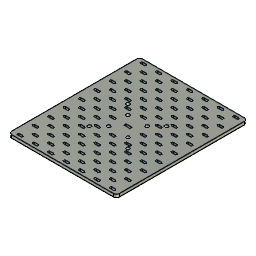
SkadisForUniversalScreenHolder v3 (Autodesk Fusion 360 design; units mm, degrees)
Autodesk Fusion 360 part; units mm, degrees
(part 1 of 2)
sketch "Sketch1" plane through (0, 0, 0) normal (0, 0, 1) x (1, 0, 0)
  line L0 (8, 0) -> (272, 0)
  line L1 (280, 8) -> (280, 332)
  line L2 (272, 340) -> (8, 340)
  line L3 (0, 332) -> (0, 8)
  arc A0 (8, 340) -> (0, 332) centre (8, 332) ccw
  arc A1 (280, 332) -> (272, 340) centre (272, 332) ccw
  arc A2 (272, 0) -> (280, 8) centre (272, 8) ccw
  arc A3 (0, 8) -> (8, 0) centre (8, 8) ccw
  line L4 (8, 8) -> (272, 332) construction
  line L5 (8, 332) -> (272, 8) construction
  line L6 (190, 220) -> (90, 220) construction
  line L7 (90, 220) -> (90, 120) construction
  line L8 (90, 120) -> (190, 120) construction
  line L9 (190, 120) -> (190, 220) construction
  line L10 (190, 220) -> (90, 120) construction
  line L11 (90, 220) -> (190, 120) construction
  line L12 (165, 195) -> (115, 195) construction
  line L13 (115, 195) -> (115, 145) construction
  line L14 (115, 145) -> (165, 145) construction
  line L15 (165, 145) -> (165, 195) construction
  line L16 (165, 195) -> (115, 145) construction
  line L17 (115, 195) -> (165, 145) construction
  circle A4 centre (115, 195) radius 4.5
  circle A5 centre (165, 195) radius 4.5
  circle A6 centre (165, 145) radius 4.5
  circle A7 centre (115, 145) radius 4.5
  circle A8 centre (190, 120) radius 4.5
  circle A9 centre (90, 120) radius 4.5
  circle A10 centre (90, 220) radius 4.5
  circle A11 centre (190, 220) radius 4.5
  point P0 (280, 0)
  point P1 (0, 340)
  point P2 (140, 170)
  point P3 (140, 170)
  dimension "d1" = 280
  dimension "d2" = 340
  dimension "d3" = 8
  dimension "d4" = 100
  dimension "d5" = 100
  dimension "d6" = 50
  dimension "d7" = 50
  dimension "d10" = 9
  dimension "d11" = 9
  dimension "d12" = 9
  dimension "d13" = 9
  dimension "d14" = 9
  dimension "d15" = 9
  dimension "d16" = 9
  dimension "d17" = 9
  constraint horizontal L0
  constraint vertical L1
  constraint horizontal L2
  constraint vertical L3
  constraint coincident P1 L3
  constraint coincident P1 L2
  constraint tangent L3 A0
  constraint tangent L2 A0
  constraint tangent L2 A1
  constraint tangent L1 A1
  constraint equal A0 A1
  constraint coincident P0 L1
  constraint coincident P0 L0
  constraint tangent L1 A2
  constraint tangent L0 A2
  constraint equal A0 A2
  constraint coincident origin L0
  constraint coincident origin L3
  constraint tangent L0 A3
  constraint tangent L3 A3
  constraint equal A0 A3
  constraint coincident A3.centre L4.start
  constraint coincident A1.centre L4.end
  constraint coincident A0.centre L5.start
  constraint coincident A2.centre L5.end
  constraint horizontal L6
  constraint perpendicular L6 L7
  constraint parallel L6 L8
  constraint parallel L7 L9
  constraint coincident L10 P3
  constraint coincident L11 P3
  constraint midpoint L4 P3
  constraint horizontal L12
  constraint perpendicular L12 L13
  constraint parallel L12 L14
  constraint parallel L13 L15
  constraint coincident L16 P3
  constraint coincident L17 P3
  constraint coincident P3 P2
  constraint coincident L12.end L13.start
  constraint coincident L12.start L15.end
  constraint coincident L14.end L15.start
  constraint coincident L13.end L14.start
  constraint coincident L8.end L9.start
  constraint coincident L7.end L8.start
  constraint coincident L6.end L7.start
  constraint coincident L6.start L9.end
  constraint equal A5 A11
  constraint equal A5 A6
  constraint equal A6 A7
  constraint equal A7 A10
  constraint equal A9 A10
  constraint equal A8 A9
  measures "d1" distance of origin P0
  measures "d2" distance of origin P1
  measures "d3" radius of A0
  measures "d4" distance of L7.end L8.end
  measures "d5" distance of L6.end L7.end
  measures "d6" distance of L13.end L14.end
  measures "d7" distance of L12.end L13.end
  measures "d10" diameter of A10
  measures "d11" diameter of A11
  measures "d12" diameter of A5
  measures "d13" diameter of A6
  measures "d14" diameter of A8
  measures "d15" diameter of A7
  measures "d16" diameter of A9
  measures "d17" diameter of A4
extrude "Extrude1" add sketch "Sketch1" along normal blind 8
sketch "Sketch2" plane through (0, 0, 8) normal (0, 0, 1) x (-1, 0, 0)
  circle A0 centre (-165, -145) radius 4.5
  circle A1 centre (-90, -120) radius 4.5
  circle A2 centre (-165, -195) radius 4.5
  circle A3 centre (-190, -120) radius 4.5
  circle A4 centre (-115, -145) radius 4.5
  circle A5 centre (-190, -220) radius 4.5
  circle A6 centre (-90, -220) radius 4.5
  circle A7 centre (-115, -195) radius 4.5
  line L0 (-147.5, -167.5) -> (-132.5, -167.5)
  line L1 (-132.5, -167.5) -> (-132.5, -172.5)
  line L2 (-132.5, -172.5) -> (-147.5, -172.5)
  line L3 (-147.5, -172.5) -> (-147.5, -167.5)
  line L4 (-147.5, -167.5) -> (-132.5, -172.5) construction
  line L5 (-132.5, -167.5) -> (-147.5, -172.5) construction
  line L6 (-135, -167.5) -> (-145, -167.5)
  arc A8 (-145, -167.5) -> (-145, -172.5) centre (-145, -170) ccw
  line L7 (-145, -172.5) -> (-135, -172.5)
  arc A9 (-135, -172.5) -> (-135, -167.5) centre (-135, -170) ccw
  line L8 (-132.5, -170) -> (-147.5, -170) construction
  arc A10 (-255, -332.5) -> (-255, -327.5) centre (-255, -330) ccw
  line L9 (-255, -327.5) -> (-265, -327.5)
  arc A11 (-265, -327.5) -> (-265, -332.5) centre (-265, -330) ccw
  line L10 (-265, -332.5) -> (-255, -332.5)
  arc A12 (-215, -332.5) -> (-215, -327.5) centre (-215, -330) ccw
  line L11 (-215, -327.5) -> (-225, -327.5)
  arc A13 (-225, -327.5) -> (-225, -332.5) centre (-225, -330) ccw
  line L12 (-225, -332.5) -> (-215, -332.5)
  arc A14 (-175, -332.5) -> (-175, -327.5) centre (-175, -330) ccw
  line L13 (-175, -327.5) -> (-185, -327.5)
  arc A15 (-185, -327.5) -> (-185, -332.5) centre (-185, -330) ccw
  line L14 (-185, -332.5) -> (-175, -332.5)
  arc A16 (-135, -332.5) -> (-135, -327.5) centre (-135, -330) ccw
  line L15 (-135, -327.5) -> (-145, -327.5)
  arc A17 (-145, -327.5) -> (-145, -332.5) centre (-145, -330) ccw
  line L16 (-145, -332.5) -> (-135, -332.5)
  arc A18 (-95, -332.5) -> (-95, -327.5) centre (-95, -330) ccw
  line L17 (-95, -327.5) -> (-105, -327.5)
  arc A19 (-105, -327.5) -> (-105, -332.5) centre (-105, -330) ccw
  line L18 (-105, -332.5) -> (-95, -332.5)
  arc A20 (-55, -332.5) -> (-55, -327.5) centre (-55, -330) ccw
  line L19 (-55, -327.5) -> (-65, -327.5)
  arc A21 (-65, -327.5) -> (-65, -332.5) centre (-65, -330) ccw
  line L20 (-65, -332.5) -> (-55, -332.5)
  arc A22 (-15, -332.5) -> (-15, -327.5) centre (-15, -330) ccw
  line L21 (-15, -327.5) -> (-25, -327.5)
  arc A23 (-25, -327.5) -> (-25, -332.5) centre (-25, -330) ccw
  line L22 (-25, -332.5) -> (-15, -332.5)
  arc A24 (-255, -292.5) -> (-255, -287.5) centre (-255, -290) ccw
  line L23 (-255, -287.5) -> (-265, -287.5)
  arc A25 (-265, -287.5) -> (-265, -292.5) centre (-265, -290) ccw
  line L24 (-265, -292.5) -> (-255, -292.5)
  arc A26 (-215, -292.5) -> (-215, -287.5) centre (-215, -290) ccw
  line L25 (-215, -287.5) -> (-225, -287.5)
  arc A27 (-225, -287.5) -> (-225, -292.5) centre (-225, -290) ccw
  line L26 (-225, -292.5) -> (-215, -292.5)
  arc A28 (-175, -292.5) -> (-175, -287.5) centre (-175, -290) ccw
  line L27 (-175, -287.5) -> (-185, -287.5)
  arc A29 (-185, -287.5) -> (-185, -292.5) centre (-185, -290) ccw
  line L28 (-185, -292.5) -> (-175, -292.5)
  arc A30 (-135, -292.5) -> (-135, -287.5) centre (-135, -290) ccw
  line L29 (-135, -287.5) -> (-145, -287.5)
  arc A31 (-145, -287.5) -> (-145, -292.5) centre (-145, -290) ccw
  line L30 (-145, -292.5) -> (-135, -292.5)
  arc A32 (-95, -292.5) -> (-95, -287.5) centre (-95, -290) ccw
  line L31 (-95, -287.5) -> (-105, -287.5)
  arc A33 (-105, -287.5) -> (-105, -292.5) centre (-105, -290) ccw
  line L32 (-105, -292.5) -> (-95, -292.5)
  arc A34 (-55, -292.5) -> (-55, -287.5) centre (-55, -290) ccw
  line L33 (-55, -287.5) -> (-65, -287.5)
  arc A35 (-65, -287.5) -> (-65, -292.5) centre (-65, -290) ccw
  line L34 (-65, -292.5) -> (-55, -292.5)
  arc A36 (-15, -292.5) -> (-15, -287.5) centre (-15, -290) ccw
  line L35 (-15, -287.5) -> (-25, -287.5)
  arc A37 (-25, -287.5) -> (-25, -292.5) centre (-25, -290) ccw
  line L36 (-25, -292.5) -> (-15, -292.5)
  arc A38 (-255, -252.5) -> (-255, -247.5) centre (-255, -250) ccw
  line L37 (-255, -247.5) -> (-265, -247.5)
  arc A39 (-265, -247.5) -> (-265, -252.5) centre (-265, -250) ccw
  line L38 (-265, -252.5) -> (-255, -252.5)
  arc A40 (-215, -252.5) -> (-215, -247.5) centre (-215, -250) ccw
  line L39 (-215, -247.5) -> (-225, -247.5)
  arc A41 (-225, -247.5) -> (-225, -252.5) centre (-225, -250) ccw
  line L40 (-225, -252.5) -> (-215, -252.5)
  arc A42 (-175, -252.5) -> (-175, -247.5) centre (-175, -250) ccw
  line L41 (-175, -247.5) -> (-185, -247.5)
  arc A43 (-185, -247.5) -> (-185, -252.5) centre (-185, -250) ccw
  line L42 (-185, -252.5) -> (-175, -252.5)
  arc A44 (-135, -252.5) -> (-135, -247.5) centre (-135, -250) ccw
  line L43 (-135, -247.5) -> (-145, -247.5)
  arc A45 (-145, -247.5) -> (-145, -252.5) centre (-145, -250) ccw
  line L44 (-145, -252.5) -> (-135, -252.5)
  arc A46 (-95, -252.5) -> (-95, -247.5) centre (-95, -250) ccw
  line L45 (-95, -247.5) -> (-105, -247.5)
  arc A47 (-105, -247.5) -> (-105, -252.5) centre (-105, -250) ccw
  line L46 (-105, -252.5) -> (-95, -252.5)
  arc A48 (-55, -252.5) -> (-55, -247.5) centre (-55, -250) ccw
  line L47 (-55, -247.5) -> (-65, -247.5)
  arc A49 (-65, -247.5) -> (-65, -252.5) centre (-65, -250) ccw
  line L48 (-65, -252.5) -> (-55, -252.5)
  arc A50 (-15, -252.5) -> (-15, -247.5) centre (-15, -250) ccw
  line L49 (-15, -247.5) -> (-25, -247.5)
  arc A51 (-25, -247.5) -> (-25, -252.5) centre (-25, -250) ccw
  line L50 (-25, -252.5) -> (-15, -252.5)
  arc A52 (-255, -212.5) -> (-255, -207.5) centre (-255, -210) ccw
  line L51 (-255, -207.5) -> (-265, -207.5)
  arc A53 (-265, -207.5) -> (-265, -212.5) centre (-265, -210) ccw
  line L52 (-265, -212.5) -> (-255, -212.5)
  arc A54 (-215, -212.5) -> (-215, -207.5) centre (-215, -210) ccw
  line L53 (-215, -207.5) -> (-225, -207.5)
  arc A55 (-225, -207.5) -> (-225, -212.5) centre (-225, -210) ccw
  line L54 (-225, -212.5) -> (-215, -212.5)
  arc A56 (-175, -212.5) -> (-175, -207.5) centre (-175, -210) ccw
  line L55 (-175, -207.5) -> (-185, -207.5)
  arc A57 (-185, -207.5) -> (-185, -212.5) centre (-185, -210) ccw
  line L56 (-185, -212.5) -> (-175, -212.5)
  arc A58 (-135, -212.5) -> (-135, -207.5) centre (-135, -210) ccw
  line L57 (-135, -207.5) -> (-145, -207.5)
  arc A59 (-145, -207.5) -> (-145, -212.5) centre (-145, -210) ccw
  line L58 (-145, -212.5) -> (-135, -212.5)
  arc A60 (-95, -212.5) -> (-95, -207.5) centre (-95, -210) ccw
  line L59 (-95, -207.5) -> (-105, -207.5)
  arc A61 (-105, -207.5) -> (-105, -212.5) centre (-105, -210) ccw
  line L60 (-105, -212.5) -> (-95, -212.5)
  arc A62 (-55, -212.5) -> (-55, -207.5) centre (-55, -210) ccw
  line L61 (-55, -207.5) -> (-65, -207.5)
  arc A63 (-65, -207.5) -> (-65, -212.5) centre (-65, -210) ccw
  line L62 (-65, -212.5) -> (-55, -212.5)
  arc A64 (-15, -212.5) -> (-15, -207.5) centre (-15, -210) ccw
  line L63 (-15, -207.5) -> (-25, -207.5)
  arc A65 (-25, -207.5) -> (-25, -212.5) centre (-25, -210) ccw
  line L64 (-25, -212.5) -> (-15, -212.5)
  arc A66 (-255, -172.5) -> (-255, -167.5) centre (-255, -170) ccw
  line L65 (-255, -167.5) -> (-265, -167.5)
  arc A67 (-265, -167.5) -> (-265, -172.5) centre (-265, -170) ccw
  line L66 (-265, -172.5) -> (-255, -172.5)
  arc A68 (-215, -172.5) -> (-215, -167.5) centre (-215, -170) ccw
  line L67 (-215, -167.5) -> (-225, -167.5)
  arc A69 (-225, -167.5) -> (-225, -172.5) centre (-225, -170) ccw
  line L68 (-225, -172.5) -> (-215, -172.5)
  arc A70 (-175, -172.5) -> (-175, -167.5) centre (-175, -170) ccw
  line L69 (-175, -167.5) -> (-185, -167.5)
  arc A71 (-185, -167.5) -> (-185, -172.5) centre (-185, -170) ccw
  line L70 (-185, -172.5) -> (-175, -172.5)
  arc A72 (-95, -172.5) -> (-95, -167.5) centre (-95, -170) ccw
  line L71 (-95, -167.5) -> (-105, -167.5)
  arc A73 (-105, -167.5) -> (-105, -172.5) centre (-105, -170) ccw
  line L72 (-105, -172.5) -> (-95, -172.5)
  arc A74 (-55, -172.5) -> (-55, -167.5) centre (-55, -170) ccw
  line L73 (-55, -167.5) -> (-65, -167.5)
  arc A75 (-65, -167.5) -> (-65, -172.5) centre (-65, -170) ccw
  line L74 (-65, -172.5) -> (-55, -172.5)
  arc A76 (-15, -172.5) -> (-15, -167.5) centre (-15, -170) ccw
  line L75 (-15, -167.5) -> (-25, -167.5)
  arc A77 (-25, -167.5) -> (-25, -172.5) centre (-25, -170) ccw
  line L76 (-25, -172.5) -> (-15, -172.5)
  arc A78 (-255, -132.5) -> (-255, -127.5) centre (-255, -130) ccw
  line L77 (-255, -127.5) -> (-265, -127.5)
  arc A79 (-265, -127.5) -> (-265, -132.5) centre (-265, -130) ccw
  line L78 (-265, -132.5) -> (-255, -132.5)
  arc A80 (-215, -132.5) -> (-215, -127.5) centre (-215, -130) ccw
  line L79 (-215, -127.5) -> (-225, -127.5)
  arc A81 (-225, -127.5) -> (-225, -132.5) centre (-225, -130) ccw
  line L80 (-225, -132.5) -> (-215, -132.5)
  arc A82 (-175, -132.5) -> (-175, -127.5) centre (-175, -130) ccw
  line L81 (-175, -127.5) -> (-185, -127.5)
  arc A83 (-185, -127.5) -> (-185, -132.5) centre (-185, -130) ccw
  line L82 (-185, -132.5) -> (-175, -132.5)
  arc A84 (-135, -132.5) -> (-135, -127.5) centre (-135, -130) ccw
  line L83 (-135, -127.5) -> (-145, -127.5)
  arc A85 (-145, -127.5) -> (-145, -132.5) centre (-145, -130) ccw
  line L84 (-145, -132.5) -> (-135, -132.5)
  arc A86 (-95, -132.5) -> (-95, -127.5) centre (-95, -130) ccw
  line L85 (-95, -127.5) -> (-105, -127.5)
  arc A87 (-105, -127.5) -> (-105, -132.5) centre (-105, -130) ccw
  line L86 (-105, -132.5) -> (-95, -132.5)
  arc A88 (-55, -132.5) -> (-55, -127.5) centre (-55, -130) ccw
  line L87 (-55, -127.5) -> (-65, -127.5)
  arc A89 (-65, -127.5) -> (-65, -132.5) centre (-65, -130) ccw
  line L88 (-65, -132.5) -> (-55, -132.5)
  arc A90 (-15, -132.5) -> (-15, -127.5) centre (-15, -130) ccw
  line L89 (-15, -127.5) -> (-25, -127.5)
  arc A91 (-25, -127.5) -> (-25, -132.5) centre (-25, -130) ccw
  line L90 (-25, -132.5) -> (-15, -132.5)
  arc A92 (-255, -92.5) -> (-255, -87.5) centre (-255, -90) ccw
  line L91 (-255, -87.5) -> (-265, -87.5)
  arc A93 (-265, -87.5) -> (-265, -92.5) centre (-265, -90) ccw
  line L92 (-265, -92.5) -> (-255, -92.5)
  arc A94 (-215, -92.5) -> (-215, -87.5) centre (-215, -90) ccw
  line L93 (-215, -87.5) -> (-225, -87.5)
  arc A95 (-225, -87.5) -> (-225, -92.5) centre (-225, -90) ccw
  line L94 (-225, -92.5) -> (-215, -92.5)
  arc A96 (-175, -92.5) -> (-175, -87.5) centre (-175, -90) ccw
  line L95 (-175, -87.5) -> (-185, -87.5)
  arc A97 (-185, -87.5) -> (-185, -92.5) centre (-185, -90) ccw
  line L96 (-185, -92.5) -> (-175, -92.5)
  arc A98 (-135, -92.5) -> (-135, -87.5) centre (-135, -90) ccw
  line L97 (-135, -87.5) -> (-145, -87.5)
  arc A99 (-145, -87.5) -> (-145, -92.5) centre (-145, -90) ccw
  line L98 (-145, -92.5) -> (-135, -92.5)
  arc A100 (-95, -92.5) -> (-95, -87.5) centre (-95, -90) ccw
  line L99 (-95, -87.5) -> (-105, -87.5)
  arc A101 (-105, -87.5) -> (-105, -92.5) centre (-105, -90) ccw
  line L100 (-105, -92.5) -> (-95, -92.5)
  arc A102 (-55, -92.5) -> (-55, -87.5) centre (-55, -90) ccw
  line L101 (-55, -87.5) -> (-65, -87.5)
  arc A103 (-65, -87.5) -> (-65, -92.5) centre (-65, -90) ccw
  line L102 (-65, -92.5) -> (-55, -92.5)
  arc A104 (-15, -92.5) -> (-15, -87.5) centre (-15, -90) ccw
  line L103 (-15, -87.5) -> (-25, -87.5)
  arc A105 (-25, -87.5) -> (-25, -92.5) centre (-25, -90) ccw
  line L104 (-25, -92.5) -> (-15, -92.5)
  arc A106 (-255, -52.5) -> (-255, -47.5) centre (-255, -50) ccw
  line L105 (-255, -47.5) -> (-265, -47.5)
  arc A107 (-265, -47.5) -> (-265, -52.5) centre (-265, -50) ccw
  line L106 (-265, -52.5) -> (-255, -52.5)
  arc A108 (-215, -52.5) -> (-215, -47.5) centre (-215, -50) ccw
  line L107 (-215, -47.5) -> (-225, -47.5)
  arc A109 (-225, -47.5) -> (-225, -52.5) centre (-225, -50) ccw
  line L108 (-225, -52.5) -> (-215, -52.5)
  arc A110 (-175, -52.5) -> (-175, -47.5) centre (-175, -50) ccw
  line L109 (-175, -47.5) -> (-185, -47.5)
  arc A111 (-185, -47.5) -> (-185, -52.5) centre (-185, -50) ccw
  line L110 (-185, -52.5) -> (-175, -52.5)
  arc A112 (-135, -52.5) -> (-135, -47.5) centre (-135, -50) ccw
  line L111 (-135, -47.5) -> (-145, -47.5)
  arc A113 (-145, -47.5) -> (-145, -52.5) centre (-145, -50) ccw
  line L112 (-145, -52.5) -> (-135, -52.5)
  arc A114 (-95, -52.5) -> (-95, -47.5) centre (-95, -50) ccw
  line L113 (-95, -47.5) -> (-105, -47.5)
  arc A115 (-105, -47.5) -> (-105, -52.5) centre (-105, -50) ccw
  line L114 (-105, -52.5) -> (-95, -52.5)
  arc A116 (-55, -52.5) -> (-55, -47.5) centre (-55, -50) ccw
  line L115 (-55, -47.5) -> (-65, -47.5)
  arc A117 (-65, -47.5) -> (-65, -52.5) centre (-65, -50) ccw
  line L116 (-65, -52.5) -> (-55, -52.5)
  arc A118 (-15, -52.5) -> (-15, -47.5) centre (-15, -50) ccw
  line L117 (-15, -47.5) -> (-25, -47.5)
  arc A119 (-25, -47.5) -> (-25, -52.5) centre (-25, -50) ccw
  line L118 (-25, -52.5) -> (-15, -52.5)
  arc A120 (-255, -12.5) -> (-255, -7.5) centre (-255, -10) ccw
  line L119 (-255, -7.5) -> (-265, -7.5)
  arc A121 (-265, -7.5) -> (-265, -12.5) centre (-265, -10) ccw
  line L120 (-265, -12.5) -> (-255, -12.5)
  arc A122 (-215, -12.5) -> (-215, -7.5) centre (-215, -10) ccw
  line L121 (-215, -7.5) -> (-225, -7.5)
  arc A123 (-225, -7.5) -> (-225, -12.5) centre (-225, -10) ccw
  line L122 (-225, -12.5) -> (-215, -12.5)
  arc A124 (-175, -12.5) -> (-175, -7.5) centre (-175, -10) ccw
  line L123 (-175, -7.5) -> (-185, -7.5)
  arc A125 (-185, -7.5) -> (-185, -12.5) centre (-185, -10) ccw
  line L124 (-185, -12.5) -> (-175, -12.5)
  arc A126 (-135, -12.5) -> (-135, -7.5) centre (-135, -10) ccw
  line L125 (-135, -7.5) -> (-145, -7.5)
  arc A127 (-145, -7.5) -> (-145, -12.5) centre (-145, -10) ccw
  line L126 (-145, -12.5) -> (-135, -12.5)
  arc A128 (-95, -12.5) -> (-95, -7.5) centre (-95, -10) ccw
  line L127 (-95, -7.5) -> (-105, -7.5)
  arc A129 (-105, -7.5) -> (-105, -12.5) centre (-105, -10) ccw
  line L128 (-105, -12.5) -> (-95, -12.5)
  arc A130 (-55, -12.5) -> (-55, -7.5) centre (-55, -10) ccw
  line L129 (-55, -7.5) -> (-65, -7.5)
  arc A131 (-65, -7.5) -> (-65, -12.5) centre (-65, -10) ccw
  line L130 (-65, -12.5) -> (-55, -12.5)
  arc A132 (-15, -12.5) -> (-15, -7.5) centre (-15, -10) ccw
  line L131 (-15, -7.5) -> (-25, -7.5)
  arc A133 (-25, -7.5) -> (-25, -12.5) centre (-25, -10) ccw
  line L132 (-25, -12.5) -> (-15, -12.5)
  line L133 (-35, -27.5) -> (-45, -27.5)
  arc A134 (-45, -27.5) -> (-45, -32.5) centre (-45, -30) ccw
  line L134 (-45, -32.5) -> (-35, -32.5)
  arc A135 (-35, -32.5) -> (-35, -27.5) centre (-35, -30) ccw
  line L135 (-85, -32.5) -> (-75, -32.5)
  arc A136 (-75, -32.5) -> (-75, -27.5) centre (-75, -30) ccw
  line L136 (-75, -27.5) -> (-85, -27.5)
  arc A137 (-85, -27.5) -> (-85, -32.5) centre (-85, -30) ccw
  line L137 (-125, -32.5) -> (-115, -32.5)
  arc A138 (-115, -32.5) -> (-115, -27.5) centre (-115, -30) ccw
  line L138 (-115, -27.5) -> (-125, -27.5)
  arc A139 (-125, -27.5) -> (-125, -32.5) centre (-125, -30) ccw
  line L139 (-165, -32.5) -> (-155, -32.5)
  arc A140 (-155, -32.5) -> (-155, -27.5) centre (-155, -30) ccw
  line L140 (-155, -27.5) -> (-165, -27.5)
  arc A141 (-165, -27.5) -> (-165, -32.5) centre (-165, -30) ccw
  line L141 (-205, -32.5) -> (-195, -32.5)
  arc A142 (-195, -32.5) -> (-195, -27.5) centre (-195, -30) ccw
  line L142 (-195, -27.5) -> (-205, -27.5)
  arc A143 (-205, -27.5) -> (-205, -32.5) centre (-205, -30) ccw
  line L143 (-245, -32.5) -> (-235, -32.5)
  arc A144 (-235, -32.5) -> (-235, -27.5) centre (-235, -30) ccw
  line L144 (-235, -27.5) -> (-245, -27.5)
  arc A145 (-245, -27.5) -> (-245, -32.5) centre (-245, -30) ccw
  line L145 (-45, -72.5) -> (-35, -72.5)
  arc A146 (-35, -72.5) -> (-35, -67.5) centre (-35, -70) ccw
  line L146 (-35, -67.5) -> (-45, -67.5)
  arc A147 (-45, -67.5) -> (-45, -72.5) centre (-45, -70) ccw
  line L147 (-85, -72.5) -> (-75, -72.5)
  arc A148 (-75, -72.5) -> (-75, -67.5) centre (-75, -70) ccw
  line L148 (-75, -67.5) -> (-85, -67.5)
  arc A149 (-85, -67.5) -> (-85, -72.5) centre (-85, -70) ccw
  line L149 (-125, -72.5) -> (-115, -72.5)
  arc A150 (-115, -72.5) -> (-115, -67.5) centre (-115, -70) ccw
  line L150 (-115, -67.5) -> (-125, -67.5)
  arc A151 (-125, -67.5) -> (-125, -72.5) centre (-125, -70) ccw
  line L151 (-165, -72.5) -> (-155, -72.5)
  arc A152 (-155, -72.5) -> (-155, -67.5) centre (-155, -70) ccw
  line L152 (-155, -67.5) -> (-165, -67.5)
  arc A153 (-165, -67.5) -> (-165, -72.5) centre (-165, -70) ccw
  line L153 (-205, -72.5) -> (-195, -72.5)
  arc A154 (-195, -72.5) -> (-195, -67.5) centre (-195, -70) ccw
  line L154 (-195, -67.5) -> (-205, -67.5)
  arc A155 (-205, -67.5) -> (-205, -72.5) centre (-205, -70) ccw
  line L155 (-245, -72.5) -> (-235, -72.5)
  arc A156 (-235, -72.5) -> (-235, -67.5) centre (-235, -70) ccw
  line L156 (-235, -67.5) -> (-245, -67.5)
  arc A157 (-245, -67.5) -> (-245, -72.5) centre (-245, -70) ccw
  line L157 (-45, -112.5) -> (-35, -112.5)
  arc A158 (-35, -112.5) -> (-35, -107.5) centre (-35, -110) ccw
  line L158 (-35, -107.5) -> (-45, -107.5)
  arc A159 (-45, -107.5) -> (-45, -112.5) centre (-45, -110) ccw
  line L159 (-85, -112.5) -> (-75, -112.5)
  arc A160 (-75, -112.5) -> (-75, -107.5) centre (-75, -110) ccw
  line L160 (-75, -107.5) -> (-85, -107.5)
  arc A161 (-85, -107.5) -> (-85, -112.5) centre (-85, -110) ccw
  line L161 (-125, -112.5) -> (-115, -112.5)
  arc A162 (-115, -112.5) -> (-115, -107.5) centre (-115, -110) ccw
  line L162 (-115, -107.5) -> (-125, -107.5)
  arc A163 (-125, -107.5) -> (-125, -112.5) centre (-125, -110) ccw
  line L163 (-165, -112.5) -> (-155, -112.5)
  arc A164 (-155, -112.5) -> (-155, -107.5) centre (-155, -110) ccw
  line L164 (-155, -107.5) -> (-165, -107.5)
  arc A165 (-165, -107.5) -> (-165, -112.5) centre (-165, -110) ccw
  line L165 (-205, -112.5) -> (-195, -112.5)
  arc A166 (-195, -112.5) -> (-195, -107.5) centre (-195, -110) ccw
  line L166 (-195, -107.5) -> (-205, -107.5)
  arc A167 (-205, -107.5) -> (-205, -112.5) centre (-205, -110) ccw
  line L167 (-245, -112.5) -> (-235, -112.5)
  arc A168 (-235, -112.5) -> (-235, -107.5) centre (-235, -110) ccw
  line L168 (-235, -107.5) -> (-245, -107.5)
  arc A169 (-245, -107.5) -> (-245, -112.5) centre (-245, -110) ccw
  line L169 (-45, -152.5) -> (-35, -152.5)
  arc A170 (-35, -152.5) -> (-35, -147.5) centre (-35, -150) ccw
  line L170 (-35, -147.5) -> (-45, -147.5)
  arc A171 (-45, -147.5) -> (-45, -152.5) centre (-45, -150) ccw
  line L171 (-85, -152.5) -> (-75, -152.5)
  arc A172 (-75, -152.5) -> (-75, -147.5) centre (-75, -150) ccw
  line L172 (-75, -147.5) -> (-85, -147.5)
  arc A173 (-85, -147.5) -> (-85, -152.5) centre (-85, -150) ccw
  line L173 (-205, -152.5) -> (-195, -152.5)
  arc A174 (-195, -152.5) -> (-195, -147.5) centre (-195, -150) ccw
  line L174 (-195, -147.5) -> (-205, -147.5)
  arc A175 (-205, -147.5) -> (-205, -152.5) centre (-205, -150) ccw
  line L175 (-245, -152.5) -> (-235, -152.5)
  arc A176 (-235, -152.5) -> (-235, -147.5) centre (-235, -150) ccw
  line L176 (-235, -147.5) -> (-245, -147.5)
  arc A177 (-245, -147.5) -> (-245, -152.5) centre (-245, -150) ccw
  line L177 (-45, -192.5) -> (-35, -192.5)
  arc A178 (-35, -192.5) -> (-35, -187.5) centre (-35, -190) ccw
  line L178 (-35, -187.5) -> (-45, -187.5)
  arc A179 (-45, -187.5) -> (-45, -192.5) centre (-45, -190) ccw
  line L179 (-85, -192.5) -> (-75, -192.5)
  arc A180 (-75, -192.5) -> (-75, -187.5) centre (-75, -190) ccw
  line L180 (-75, -187.5) -> (-85, -187.5)
  arc A181 (-85, -187.5) -> (-85, -192.5) centre (-85, -190) ccw
  line L181 (-205, -192.5) -> (-195, -192.5)
  arc A182 (-195, -192.5) -> (-195, -187.5) centre (-195, -190) ccw
  line L182 (-195, -187.5) -> (-205, -187.5)
  arc A183 (-205, -187.5) -> (-205, -192.5) centre (-205, -190) ccw
  line L183 (-245, -192.5) -> (-235, -192.5)
  arc A184 (-235, -192.5) -> (-235, -187.5) centre (-235, -190) ccw
  line L184 (-235, -187.5) -> (-245, -187.5)
  arc A185 (-245, -187.5) -> (-245, -192.5) centre (-245, -190) ccw
  line L185 (-45, -232.5) -> (-35, -232.5)
  arc A186 (-35, -232.5) -> (-35, -227.5) centre (-35, -230) ccw
  line L186 (-35, -227.5) -> (-45, -227.5)
  arc A187 (-45, -227.5) -> (-45, -232.5) centre (-45, -230) ccw
  line L187 (-85, -232.5) -> (-75, -232.5)
  arc A188 (-75, -232.5) -> (-75, -227.5) centre (-75, -230) ccw
  line L188 (-75, -227.5) -> (-85, -227.5)
  arc A189 (-85, -227.5) -> (-85, -232.5) centre (-85, -230) ccw
  line L189 (-125, -232.5) -> (-115, -232.5)
  arc A190 (-115, -232.5) -> (-115, -227.5) centre (-115, -230) ccw
  line L190 (-115, -227.5) -> (-125, -227.5)
  arc A191 (-125, -227.5) -> (-125, -232.5) centre (-125, -230) ccw
  line L191 (-165, -232.5) -> (-155, -232.5)
  arc A192 (-155, -232.5) -> (-155, -227.5) centre (-155, -230) ccw
  line L192 (-155, -227.5) -> (-165, -227.5)
  arc A193 (-165, -227.5) -> (-165, -232.5) centre (-165, -230) ccw
  line L193 (-205, -232.5) -> (-195, -232.5)
  arc A194 (-195, -232.5) -> (-195, -227.5) centre (-195, -230) ccw
  line L194 (-195, -227.5) -> (-205, -227.5)
  arc A195 (-205, -227.5) -> (-205, -232.5) centre (-205, -230) ccw
  line L195 (-245, -232.5) -> (-235, -232.5)
  arc A196 (-235, -232.5) -> (-235, -227.5) centre (-235, -230) ccw
  line L196 (-235, -227.5) -> (-245, -227.5)
  arc A197 (-245, -227.5) -> (-245, -232.5) centre (-245, -230) ccw
  line L197 (-45, -272.5) -> (-35, -272.5)
  arc A198 (-35, -272.5) -> (-35, -267.5) centre (-35, -270) ccw
  line L198 (-35, -267.5) -> (-45, -267.5)
  arc A199 (-45, -267.5) -> (-45, -272.5) centre (-45, -270) ccw
  line L199 (-85, -272.5) -> (-75, -272.5)
  arc A200 (-75, -272.5) -> (-75, -267.5) centre (-75, -270) ccw
  line L200 (-75, -267.5) -> (-85, -267.5)
  arc A201 (-85, -267.5) -> (-85, -272.5) centre (-85, -270) ccw
  line L201 (-125, -272.5) -> (-115, -272.5)
  arc A202 (-115, -272.5) -> (-115, -267.5) centre (-115, -270) ccw
  line L202 (-115, -267.5) -> (-125, -267.5)
  arc A203 (-125, -267.5) -> (-125, -272.5) centre (-125, -270) ccw
  line L203 (-165, -272.5) -> (-155, -272.5)
  arc A204 (-155, -272.5) -> (-155, -267.5) centre (-155, -270) ccw
  line L204 (-155, -267.5) -> (-165, -267.5)
  arc A205 (-165, -267.5) -> (-165, -272.5) centre (-165, -270) ccw
  line L205 (-205, -272.5) -> (-195, -272.5)
  arc A206 (-195, -272.5) -> (-195, -267.5) centre (-195, -270) ccw
  line L206 (-195, -267.5) -> (-205, -267.5)
  arc A207 (-205, -267.5) -> (-205, -272.5) centre (-205, -270) ccw
  line L207 (-245, -272.5) -> (-235, -272.5)
  arc A208 (-235, -272.5) -> (-235, -267.5) centre (-235, -270) ccw
  line L208 (-235, -267.5) -> (-245, -267.5)
  arc A209 (-245, -267.5) -> (-245, -272.5) centre (-245, -270) ccw
  line L209 (-45, -312.5) -> (-35, -312.5)
  arc A210 (-35, -312.5) -> (-35, -307.5) centre (-35, -310) ccw
  line L210 (-35, -307.5) -> (-45, -307.5)
  arc A211 (-45, -307.5) -> (-45, -312.5) centre (-45, -310) ccw
  line L211 (-85, -312.5) -> (-75, -312.5)
  arc A212 (-75, -312.5) -> (-75, -307.5) centre (-75, -310) ccw
  line L212 (-75, -307.5) -> (-85, -307.5)
  arc A213 (-85, -307.5) -> (-85, -312.5) centre (-85, -310) ccw
  line L213 (-125, -312.5) -> (-115, -312.5)
  arc A214 (-115, -312.5) -> (-115, -307.5) centre (-115, -310) ccw
  line L214 (-115, -307.5) -> (-125, -307.5)
  arc A215 (-125, -307.5) -> (-125, -312.5) centre (-125, -310) ccw
  line L215 (-165, -312.5) -> (-155, -312.5)
  arc A216 (-155, -312.5) -> (-155, -307.5) centre (-155, -310) ccw
  line L216 (-155, -307.5) -> (-165, -307.5)
  arc A217 (-165, -307.5) -> (-165, -312.5) centre (-165, -310) ccw
  line L217 (-205, -312.5) -> (-195, -312.5)
  arc A218 (-195, -312.5) -> (-195, -307.5) centre (-195, -310) ccw
  line L218 (-195, -307.5) -> (-205, -307.5)
  arc A219 (-205, -307.5) -> (-205, -312.5) centre (-205, -310) ccw
  line L219 (-245, -312.5) -> (-235, -312.5)
  arc A220 (-235, -312.5) -> (-235, -307.5) centre (-235, -310) ccw
  line L220 (-235, -307.5) -> (-245, -307.5)
  arc A221 (-245, -307.5) -> (-245, -312.5) centre (-245, -310) ccw
  point P0 (-140, -170)
  dimension "d20" = 15
  dimension "d21" = 5
  dimension "d24" = 40
  dimension "d25" = 40
  dimension "d28" = -40
  dimension "d29" = -40
  constraint horizontal L0
  constraint perpendicular L0 L1
  constraint parallel L0 L2
  constraint parallel L1 L3
  constraint coincident L4 P0
  constraint coincident L5 P0
  constraint tangent L6 A8
  constraint tangent A8 L7
  constraint parallel L6 L7
  constraint tangent L7 A9
  constraint tangent L6 A9
  constraint midpoint A9 L8.start
  constraint midpoint A8 L8.end
  constraint midpoint L3 L8.end
  constraint perpendicular L3 L8
  constraint midpoint L1 L8.start
  measures "d20" distance of L1.end L2.end
  measures "d21" distance of L0.end L1.end
extrude "Extrude2" cut sketch "Sketch2" against normal blind 20
sketch "Sketch3" plane through (0, 0, 8) normal (0, 0, 1) x (-1, 0, 0)
  arc A0 (-135, -12.5) -> (-135, -7.5) centre (-135, -10) ccw
  line L0 (-135, -12.5) -> (-145, -12.5)
  arc A1 (-145, -7.5) -> (-145, -12.5) centre (-145, -10) ccw
  line L1 (-145, -7.5) -> (-135, -7.5)
  arc A2 (-255, -92.5) -> (-255, -87.5) centre (-255, -90) ccw
  line L2 (-255, -92.5) -> (-265, -92.5)
  arc A3 (-265, -87.5) -> (-265, -92.5) centre (-265, -90) ccw
  line L3 (-265, -87.5) -> (-255, -87.5)
  line L4 (-35, -192.5) -> (-45, -192.5)
  arc A4 (-45, -187.5) -> (-45, -192.5) centre (-45, -190) ccw
  line L5 (-45, -187.5) -> (-35, -187.5)
  arc A5 (-35, -192.5) -> (-35, -187.5) centre (-35, -190) ccw
  arc A6 (-135, -252.5) -> (-135, -247.5) centre (-135, -250) ccw
  line L6 (-135, -252.5) -> (-145, -252.5)
  arc A7 (-145, -247.5) -> (-145, -252.5) centre (-145, -250) ccw
  line L7 (-145, -247.5) -> (-135, -247.5)
  arc A8 (-95, -252.5) -> (-95, -247.5) centre (-95, -250) ccw
  line L8 (-95, -252.5) -> (-105, -252.5)
  arc A9 (-105, -247.5) -> (-105, -252.5) centre (-105, -250) ccw
  line L9 (-105, -247.5) -> (-95, -247.5)
  arc A10 (-15, -292.5) -> (-15, -287.5) centre (-15, -290) ccw
  line L10 (-15, -292.5) -> (-25, -292.5)
  arc A11 (-25, -287.5) -> (-25, -292.5) centre (-25, -290) ccw
  line L11 (-25, -287.5) -> (-15, -287.5)
  line L12 (-155, -72.5) -> (-165, -72.5)
  arc A12 (-165, -67.5) -> (-165, -72.5) centre (-165, -70) ccw
  line L13 (-165, -67.5) -> (-155, -67.5)
  arc A13 (-155, -72.5) -> (-155, -67.5) centre (-155, -70) ccw
  line L14 (-115, -272.5) -> (-125, -272.5)
  arc A14 (-125, -267.5) -> (-125, -272.5) centre (-125, -270) ccw
  line L15 (-125, -267.5) -> (-115, -267.5)
  arc A15 (-115, -272.5) -> (-115, -267.5) centre (-115, -270) ccw
  arc A16 (-95, -172.5) -> (-95, -167.5) centre (-95, -170) ccw
  line L16 (-95, -172.5) -> (-105, -172.5)
  arc A17 (-105, -167.5) -> (-105, -172.5) centre (-105, -170) ccw
  line L17 (-105, -167.5) -> (-95, -167.5)
  line L18 (-155, -312.5) -> (-165, -312.5)
  arc A18 (-165, -307.5) -> (-165, -312.5) centre (-165, -310) ccw
  line L19 (-165, -307.5) -> (-155, -307.5)
  arc A19 (-155, -312.5) -> (-155, -307.5) centre (-155, -310) ccw
  line L20 (-235, -232.5) -> (-245, -232.5)
  arc A20 (-245, -227.5) -> (-245, -232.5) centre (-245, -230) ccw
  line L21 (-245, -227.5) -> (-235, -227.5)
  arc A21 (-235, -232.5) -> (-235, -227.5) centre (-235, -230) ccw
  line L22 (-155, -232.5) -> (-165, -232.5)
  arc A22 (-165, -227.5) -> (-165, -232.5) centre (-165, -230) ccw
  line L23 (-165, -227.5) -> (-155, -227.5)
  arc A23 (-155, -232.5) -> (-155, -227.5) centre (-155, -230) ccw
  arc A24 (-15, -92.5) -> (-15, -87.5) centre (-15, -90) ccw
  line L24 (-15, -92.5) -> (-25, -92.5)
  arc A25 (-25, -87.5) -> (-25, -92.5) centre (-25, -90) ccw
  line L25 (-25, -87.5) -> (-15, -87.5)
  arc A26 (-55, -92.5) -> (-55, -87.5) centre (-55, -90) ccw
  line L26 (-55, -92.5) -> (-65, -92.5)
  arc A27 (-65, -87.5) -> (-65, -92.5) centre (-65, -90) ccw
  line L27 (-65, -87.5) -> (-55, -87.5)
  line L28 (-35, -272.5) -> (-45, -272.5)
  arc A28 (-45, -267.5) -> (-45, -272.5) centre (-45, -270) ccw
  line L29 (-45, -267.5) -> (-35, -267.5)
  arc A29 (-35, -272.5) -> (-35, -267.5) centre (-35, -270) ccw
  line L30 (-195, -32.5) -> (-205, -32.5)
  arc A30 (-205, -27.5) -> (-205, -32.5) centre (-205, -30) ccw
  line L31 (-205, -27.5) -> (-195, -27.5)
  arc A31 (-195, -32.5) -> (-195, -27.5) centre (-195, -30) ccw
  line L32 (-75, -272.5) -> (-85, -272.5)
  arc A32 (-85, -267.5) -> (-85, -272.5) centre (-85, -270) ccw
  line L33 (-85, -267.5) -> (-75, -267.5)
  arc A33 (-75, -272.5) -> (-75, -267.5) centre (-75, -270) ccw
  line L34 (-235, -192.5) -> (-245, -192.5)
  arc A34 (-245, -187.5) -> (-245, -192.5) centre (-245, -190) ccw
  line L35 (-245, -187.5) -> (-235, -187.5)
  arc A35 (-235, -192.5) -> (-235, -187.5) centre (-235, -190) ccw
  line L36 (-35, -112.5) -> (-45, -112.5)
  arc A36 (-45, -107.5) -> (-45, -112.5) centre (-45, -110) ccw
  line L37 (-45, -107.5) -> (-35, -107.5)
  arc A37 (-35, -112.5) -> (-35, -107.5) centre (-35, -110) ccw
  line L38 (-235, -112.5) -> (-245, -112.5)
  arc A38 (-245, -107.5) -> (-245, -112.5) centre (-245, -110) ccw
  line L39 (-245, -107.5) -> (-235, -107.5)
  arc A39 (-235, -112.5) -> (-235, -107.5) centre (-235, -110) ccw
  line L40 (-115, -232.5) -> (-125, -232.5)
  arc A40 (-125, -227.5) -> (-125, -232.5) centre (-125, -230) ccw
  line L41 (-125, -227.5) -> (-115, -227.5)
  arc A41 (-115, -232.5) -> (-115, -227.5) centre (-115, -230) ccw
  arc A42 (-55, -12.5) -> (-55, -7.5) centre (-55, -10) ccw
  line L42 (-55, -12.5) -> (-65, -12.5)
  arc A43 (-65, -7.5) -> (-65, -12.5) centre (-65, -10) ccw
  line L43 (-65, -7.5) -> (-55, -7.5)
  line L44 (-75, -232.5) -> (-85, -232.5)
  arc A44 (-85, -227.5) -> (-85, -232.5) centre (-85, -230) ccw
  line L45 (-85, -227.5) -> (-75, -227.5)
  arc A45 (-75, -232.5) -> (-75, -227.5) centre (-75, -230) ccw
  arc A46 (-175, -212.5) -> (-175, -207.5) centre (-175, -210) ccw
  line L46 (-175, -212.5) -> (-185, -212.5)
  arc A47 (-185, -207.5) -> (-185, -212.5) centre (-185, -210) ccw
  line L47 (-185, -207.5) -> (-175, -207.5)
  arc A48 (-175, -252.5) -> (-175, -247.5) centre (-175, -250) ccw
  line L48 (-175, -252.5) -> (-185, -252.5)
  arc A49 (-185, -247.5) -> (-185, -252.5) centre (-185, -250) ccw
  line L49 (-185, -247.5) -> (-175, -247.5)
  line L50 (-235, -72.5) -> (-245, -72.5)
  arc A50 (-245, -67.5) -> (-245, -72.5) centre (-245, -70) ccw
  line L51 (-245, -67.5) -> (-235, -67.5)
  arc A51 (-235, -72.5) -> (-235, -67.5) centre (-235, -70) ccw
  line L52 (-195, -112.5) -> (-205, -112.5)
  arc A52 (-205, -107.5) -> (-205, -112.5) centre (-205, -110) ccw
  line L53 (-205, -107.5) -> (-195, -107.5)
  arc A53 (-195, -112.5) -> (-195, -107.5) centre (-195, -110) ccw
  arc A54 (-255, -212.5) -> (-255, -207.5) centre (-255, -210) ccw
  line L54 (-255, -212.5) -> (-265, -212.5)
  arc A55 (-265, -207.5) -> (-265, -212.5) centre (-265, -210) ccw
  line L55 (-265, -207.5) -> (-255, -207.5)
  line L56 (-195, -72.5) -> (-205, -72.5)
  arc A56 (-205, -67.5) -> (-205, -72.5) centre (-205, -70) ccw
  line L57 (-205, -67.5) -> (-195, -67.5)
  arc A57 (-195, -72.5) -> (-195, -67.5) centre (-195, -70) ccw
  arc A58 (-255, -132.5) -> (-255, -127.5) centre (-255, -130) ccw
  line L58 (-255, -132.5) -> (-265, -132.5)
  arc A59 (-265, -127.5) -> (-265, -132.5) centre (-265, -130) ccw
  line L59 (-265, -127.5) -> (-255, -127.5)
  arc A60 (-175, -132.5) -> (-175, -127.5) centre (-175, -130) ccw
  line L60 (-175, -132.5) -> (-185, -132.5)
  arc A61 (-185, -127.5) -> (-185, -132.5) centre (-185, -130) ccw
  line L61 (-185, -127.5) -> (-175, -127.5)
  line L62 (-35, -232.5) -> (-45, -232.5)
  arc A62 (-45, -227.5) -> (-45, -232.5) centre (-45, -230) ccw
  line L63 (-45, -227.5) -> (-35, -227.5)
  arc A63 (-35, -232.5) -> (-35, -227.5) centre (-35, -230) ccw
  line L64 (-115, -112.5) -> (-125, -112.5)
  arc A64 (-125, -107.5) -> (-125, -112.5) centre (-125, -110) ccw
  line L65 (-125, -107.5) -> (-115, -107.5)
  arc A65 (-115, -112.5) -> (-115, -107.5) centre (-115, -110) ccw
  line L66 (-195, -192.5) -> (-205, -192.5)
  arc A66 (-205, -187.5) -> (-205, -192.5) centre (-205, -190) ccw
  line L67 (-205, -187.5) -> (-195, -187.5)
  arc A67 (-195, -192.5) -> (-195, -187.5) centre (-195, -190) ccw
  arc A68 (-215, -252.5) -> (-215, -247.5) centre (-215, -250) ccw
  line L68 (-215, -252.5) -> (-225, -252.5)
  arc A69 (-225, -247.5) -> (-225, -252.5) centre (-225, -250) ccw
  line L69 (-225, -247.5) -> (-215, -247.5)
  arc A70 (-135, -332.5) -> (-135, -327.5) centre (-135, -330) ccw
  line L70 (-135, -332.5) -> (-145, -332.5)
  arc A71 (-145, -327.5) -> (-145, -332.5) centre (-145, -330) ccw
  line L71 (-145, -327.5) -> (-135, -327.5)
  arc A72 (-175, -172.5) -> (-175, -167.5) centre (-175, -170) ccw
  line L72 (-175, -172.5) -> (-185, -172.5)
  arc A73 (-185, -167.5) -> (-185, -172.5) centre (-185, -170) ccw
  line L73 (-185, -167.5) -> (-175, -167.5)
  arc A74 (-95, -332.5) -> (-95, -327.5) centre (-95, -330) ccw
  line L74 (-95, -332.5) -> (-105, -332.5)
  arc A75 (-105, -327.5) -> (-105, -332.5) centre (-105, -330) ccw
  line L75 (-105, -327.5) -> (-95, -327.5)
  arc A76 (-95, -212.5) -> (-95, -207.5) centre (-95, -210) ccw
  line L76 (-95, -212.5) -> (-105, -212.5)
  arc A77 (-105, -207.5) -> (-105, -212.5) centre (-105, -210) ccw
  line L77 (-105, -207.5) -> (-95, -207.5)
  arc A78 (-95, -92.5) -> (-95, -87.5) centre (-95, -90) ccw
  line L78 (-95, -92.5) -> (-105, -92.5)
  arc A79 (-105, -87.5) -> (-105, -92.5) centre (-105, -90) ccw
  line L79 (-105, -87.5) -> (-95, -87.5)
  line L80 (-35, -152.5) -> (-45, -152.5)
  arc A80 (-45, -147.5) -> (-45, -152.5) centre (-45, -150) ccw
  line L81 (-45, -147.5) -> (-35, -147.5)
  arc A81 (-35, -152.5) -> (-35, -147.5) centre (-35, -150) ccw
  arc A82 (-175, -332.5) -> (-175, -327.5) centre (-175, -330) ccw
  line L82 (-175, -332.5) -> (-185, -332.5)
  arc A83 (-185, -327.5) -> (-185, -332.5) centre (-185, -330) ccw
  line L83 (-185, -327.5) -> (-175, -327.5)
  arc A84 (-255, -332.5) -> (-255, -327.5) centre (-255, -330) ccw
  line L84 (-255, -332.5) -> (-265, -332.5)
  arc A85 (-265, -327.5) -> (-265, -332.5) centre (-265, -330) ccw
  line L85 (-265, -327.5) -> (-255, -327.5)
  line L86 (-235, -272.5) -> (-245, -272.5)
  arc A86 (-245, -267.5) -> (-245, -272.5) centre (-245, -270) ccw
  line L87 (-245, -267.5) -> (-235, -267.5)
  arc A87 (-235, -272.5) -> (-235, -267.5) centre (-235, -270) ccw
  arc A88 (-55, -172.5) -> (-55, -167.5) centre (-55, -170) ccw
  line L88 (-55, -172.5) -> (-65, -172.5)
  arc A89 (-65, -167.5) -> (-65, -172.5) centre (-65, -170) ccw
  line L89 (-65, -167.5) -> (-55, -167.5)
  arc A90 (-15, -172.5) -> (-15, -167.5) centre (-15, -170) ccw
  line L90 (-15, -172.5) -> (-25, -172.5)
  arc A91 (-25, -167.5) -> (-25, -172.5) centre (-25, -170) ccw
  line L91 (-25, -167.5) -> (-15, -167.5)
  arc A92 (-215, -92.5) -> (-215, -87.5) centre (-215, -90) ccw
  line L92 (-215, -92.5) -> (-225, -92.5)
  arc A93 (-225, -87.5) -> (-225, -92.5) centre (-225, -90) ccw
  line L93 (-225, -87.5) -> (-215, -87.5)
  arc A94 (-15, -252.5) -> (-15, -247.5) centre (-15, -250) ccw
  line L94 (-15, -252.5) -> (-25, -252.5)
  arc A95 (-25, -247.5) -> (-25, -252.5) centre (-25, -250) ccw
  line L95 (-25, -247.5) -> (-15, -247.5)
  arc A96 (-135, -92.5) -> (-135, -87.5) centre (-135, -90) ccw
  line L96 (-135, -92.5) -> (-145, -92.5)
  arc A97 (-145, -87.5) -> (-145, -92.5) centre (-145, -90) ccw
  line L97 (-145, -87.5) -> (-135, -87.5)
  arc A98 (-55, -292.5) -> (-55, -287.5) centre (-55, -290) ccw
  line L98 (-55, -292.5) -> (-65, -292.5)
  arc A99 (-65, -287.5) -> (-65, -292.5) centre (-65, -290) ccw
  line L99 (-65, -287.5) -> (-55, -287.5)
  arc A100 (-15, -132.5) -> (-15, -127.5) centre (-15, -130) ccw
  line L100 (-15, -132.5) -> (-25, -132.5)
  arc A101 (-25, -127.5) -> (-25, -132.5) centre (-25, -130) ccw
  line L101 (-25, -127.5) -> (-15, -127.5)
  arc A102 (-175, -12.5) -> (-175, -7.5) centre (-175, -10) ccw
  line L102 (-175, -12.5) -> (-185, -12.5)
  arc A103 (-185, -7.5) -> (-185, -12.5) centre (-185, -10) ccw
  line L103 (-185, -7.5) -> (-175, -7.5)
  arc A104 (-15, -52.5) -> (-15, -47.5) centre (-15, -50) ccw
  line L104 (-15, -52.5) -> (-25, -52.5)
  arc A105 (-25, -47.5) -> (-25, -52.5) centre (-25, -50) ccw
  line L105 (-25, -47.5) -> (-15, -47.5)
  line L106 (-75, -192.5) -> (-85, -192.5)
  arc A106 (-85, -187.5) -> (-85, -192.5) centre (-85, -190) ccw
  line L107 (-85, -187.5) -> (-75, -187.5)
  arc A107 (-75, -192.5) -> (-75, -187.5) centre (-75, -190) ccw
  arc A108 (-215, -12.5) -> (-215, -7.5) centre (-215, -10) ccw
  line L108 (-215, -12.5) -> (-225, -12.5)
  arc A109 (-225, -7.5) -> (-225, -12.5) centre (-225, -10) ccw
  line L109 (-225, -7.5) -> (-215, -7.5)
  arc A110 (-175, -52.5) -> (-175, -47.5) centre (-175, -50) ccw
  line L110 (-175, -52.5) -> (-185, -52.5)
  arc A111 (-185, -47.5) -> (-185, -52.5) centre (-185, -50) ccw
  line L111 (-185, -47.5) -> (-175, -47.5)
  arc A112 (-55, -52.5) -> (-55, -47.5) centre (-55, -50) ccw
  line L112 (-55, -52.5) -> (-65, -52.5)
  arc A113 (-65, -47.5) -> (-65, -52.5) centre (-65, -50) ccw
  line L113 (-65, -47.5) -> (-55, -47.5)
  arc A114 (-95, -52.5) -> (-95, -47.5) centre (-95, -50) ccw
  line L114 (-95, -52.5) -> (-105, -52.5)
  arc A115 (-105, -47.5) -> (-105, -52.5) centre (-105, -50) ccw
  line L115 (-105, -47.5) -> (-95, -47.5)
  arc A116 (-215, -172.5) -> (-215, -167.5) centre (-215, -170) ccw
  line L116 (-215, -172.5) -> (-225, -172.5)
  arc A117 (-225, -167.5) -> (-225, -172.5) centre (-225, -170) ccw
  line L117 (-225, -167.5) -> (-215, -167.5)
  line L118 (-115, -32.5) -> (-125, -32.5)
  arc A118 (-125, -27.5) -> (-125, -32.5) centre (-125, -30) ccw
  line L119 (-125, -27.5) -> (-115, -27.5)
  arc A119 (-115, -32.5) -> (-115, -27.5) centre (-115, -30) ccw
  line L120 (-75, -312.5) -> (-85, -312.5)
  arc A120 (-85, -307.5) -> (-85, -312.5) centre (-85, -310) ccw
  line L121 (-85, -307.5) -> (-75, -307.5)
  arc A121 (-75, -312.5) -> (-75, -307.5) centre (-75, -310) ccw
  line L122 (-235, -312.5) -> (-245, -312.5)
  arc A122 (-245, -307.5) -> (-245, -312.5) centre (-245, -310) ccw
  line L123 (-245, -307.5) -> (-235, -307.5)
  arc A123 (-235, -312.5) -> (-235, -307.5) centre (-235, -310) ccw
  line L124 (-132.5, -167.5) -> (-132.5, -172.5)
  line L125 (-132.5, -172.5) -> (-147.5, -172.5)
  line L126 (-147.5, -172.5) -> (-147.5, -167.5)
  line L127 (-147.5, -167.5) -> (-132.5, -167.5)
  arc A124 (-215, -332.5) -> (-215, -327.5) centre (-215, -330) ccw
  line L128 (-215, -332.5) -> (-225, -332.5)
  arc A125 (-225, -327.5) -> (-225, -332.5) centre (-225, -330) ccw
  line L129 (-225, -327.5) -> (-215, -327.5)
  line L130 (-195, -232.5) -> (-205, -232.5)
  arc A126 (-205, -227.5) -> (-205, -232.5) centre (-205, -230) ccw
  line L131 (-205, -227.5) -> (-195, -227.5)
  arc A127 (-195, -232.5) -> (-195, -227.5) centre (-195, -230) ccw
  arc A128 (-255, -52.5) -> (-255, -47.5) centre (-255, -50) ccw
  line L132 (-255, -52.5) -> (-265, -52.5)
  arc A129 (-265, -47.5) -> (-265, -52.5) centre (-265, -50) ccw
  line L133 (-265, -47.5) -> (-255, -47.5)
  arc A130 (-15, -212.5) -> (-15, -207.5) centre (-15, -210) ccw
  line L134 (-15, -212.5) -> (-25, -212.5)
  arc A131 (-25, -207.5) -> (-25, -212.5) centre (-25, -210) ccw
  line L135 (-25, -207.5) -> (-15, -207.5)
  arc A132 (-135, -52.5) -> (-135, -47.5) centre (-135, -50) ccw
  line L136 (-135, -52.5) -> (-145, -52.5)
  arc A133 (-145, -47.5) -> (-145, -52.5) centre (-145, -50) ccw
  line L137 (-145, -47.5) -> (-135, -47.5)
  line L138 (-75, -32.5) -> (-85, -32.5)
  arc A134 (-85, -27.5) -> (-85, -32.5) centre (-85, -30) ccw
  line L139 (-85, -27.5) -> (-75, -27.5)
  arc A135 (-75, -32.5) -> (-75, -27.5) centre (-75, -30) ccw
  line L140 (-155, -32.5) -> (-165, -32.5)
  arc A136 (-165, -27.5) -> (-165, -32.5) centre (-165, -30) ccw
  line L141 (-165, -27.5) -> (-155, -27.5)
  arc A137 (-155, -32.5) -> (-155, -27.5) centre (-155, -30) ccw
  line L142 (-45, -27.5) -> (-35, -27.5)
  arc A138 (-35, -32.5) -> (-35, -27.5) centre (-35, -30) ccw
  line L143 (-35, -32.5) -> (-45, -32.5)
  arc A139 (-45, -27.5) -> (-45, -32.5) centre (-45, -30) ccw
  line L144 (-75, -112.5) -> (-85, -112.5)
  arc A140 (-85, -107.5) -> (-85, -112.5) centre (-85, -110) ccw
  line L145 (-85, -107.5) -> (-75, -107.5)
  arc A141 (-75, -112.5) -> (-75, -107.5) centre (-75, -110) ccw
  arc A142 (-255, -252.5) -> (-255, -247.5) centre (-255, -250) ccw
  line L146 (-255, -252.5) -> (-265, -252.5)
  arc A143 (-265, -247.5) -> (-265, -252.5) centre (-265, -250) ccw
  line L147 (-265, -247.5) -> (-255, -247.5)
  arc A144 (-95, -12.5) -> (-95, -7.5) centre (-95, -10) ccw
  line L148 (-95, -12.5) -> (-105, -12.5)
  arc A145 (-105, -7.5) -> (-105, -12.5) centre (-105, -10) ccw
  line L149 (-105, -7.5) -> (-95, -7.5)
  arc A146 (-95, -132.5) -> (-95, -127.5) centre (-95, -130) ccw
  line L150 (-95, -132.5) -> (-105, -132.5)
  arc A147 (-105, -127.5) -> (-105, -132.5) centre (-105, -130) ccw
  line L151 (-105, -127.5) -> (-95, -127.5)
  arc A148 (-15, -332.5) -> (-15, -327.5) centre (-15, -330) ccw
  line L152 (-15, -332.5) -> (-25, -332.5)
  arc A149 (-25, -327.5) -> (-25, -332.5) centre (-25, -330) ccw
  line L153 (-25, -327.5) -> (-15, -327.5)
  line L154 (-115, -312.5) -> (-125, -312.5)
  arc A150 (-125, -307.5) -> (-125, -312.5) centre (-125, -310) ccw
  line L155 (-125, -307.5) -> (-115, -307.5)
  arc A151 (-115, -312.5) -> (-115, -307.5) centre (-115, -310) ccw
  line L156 (-35, -72.5) -> (-45, -72.5)
  arc A152 (-45, -67.5) -> (-45, -72.5) centre (-45, -70) ccw
  line L157 (-45, -67.5) -> (-35, -67.5)
  arc A153 (-35, -72.5) -> (-35, -67.5) centre (-35, -70) ccw
  line L158 (-115, -72.5) -> (-125, -72.5)
  arc A154 (-125, -67.5) -> (-125, -72.5) centre (-125, -70) ccw
  line L159 (-125, -67.5) -> (-115, -67.5)
  arc A155 (-115, -72.5) -> (-115, -67.5) centre (-115, -70) ccw
  line L160 (-75, -72.5) -> (-85, -72.5)
  arc A156 (-85, -67.5) -> (-85, -72.5) centre (-85, -70) ccw
  line L161 (-85, -67.5) -> (-75, -67.5)
  arc A157 (-75, -72.5) -> (-75, -67.5) centre (-75, -70) ccw
  line L162 (-155, -112.5) -> (-165, -112.5)
  arc A158 (-165, -107.5) -> (-165, -112.5) centre (-165, -110) ccw
  line L163 (-165, -107.5) -> (-155, -107.5)
  arc A159 (-155, -112.5) -> (-155, -107.5) centre (-155, -110) ccw
  arc A160 (-215, -212.5) -> (-215, -207.5) centre (-215, -210) ccw
  line L164 (-215, -212.5) -> (-225, -212.5)
  arc A161 (-225, -207.5) -> (-225, -212.5) centre (-225, -210) ccw
  line L165 (-225, -207.5) -> (-215, -207.5)
  arc A162 (-215, -132.5) -> (-215, -127.5) centre (-215, -130) ccw
  line L166 (-215, -132.5) -> (-225, -132.5)
  arc A163 (-225, -127.5) -> (-225, -132.5) centre (-225, -130) ccw
  line L167 (-225, -127.5) -> (-215, -127.5)
  arc A164 (-135, -292.5) -> (-135, -287.5) centre (-135, -290) ccw
  line L168 (-135, -292.5) -> (-145, -292.5)
  arc A165 (-145, -287.5) -> (-145, -292.5) centre (-145, -290) ccw
  line L169 (-145, -287.5) -> (-135, -287.5)
  arc A166 (-135, -132.5) -> (-135, -127.5) centre (-135, -130) ccw
  line L170 (-135, -132.5) -> (-145, -132.5)
  arc A167 (-145, -127.5) -> (-145, -132.5) centre (-145, -130) ccw
  line L171 (-145, -127.5) -> (-135, -127.5)
  line L172 (-235, -152.5) -> (-245, -152.5)
  arc A168 (-245, -147.5) -> (-245, -152.5) centre (-245, -150) ccw
  line L173 (-245, -147.5) -> (-235, -147.5)
  arc A169 (-235, -152.5) -> (-235, -147.5) centre (-235, -150) ccw
  line L174 (-195, -152.5) -> (-205, -152.5)
  arc A170 (-205, -147.5) -> (-205, -152.5) centre (-205, -150) ccw
  line L175 (-205, -147.5) -> (-195, -147.5)
  arc A171 (-195, -152.5) -> (-195, -147.5) centre (-195, -150) ccw
  arc A172 (-175, -292.5) -> (-175, -287.5) centre (-175, -290) ccw
  line L176 (-175, -292.5) -> (-185, -292.5)
  arc A173 (-185, -287.5) -> (-185, -292.5) centre (-185, -290) ccw
  line L177 (-185, -287.5) -> (-175, -287.5)
  line L178 (-235, -32.5) -> (-245, -32.5)
  arc A174 (-245, -27.5) -> (-245, -32.5) centre (-245, -30) ccw
  line L179 (-245, -27.5) -> (-235, -27.5)
  arc A175 (-235, -32.5) -> (-235, -27.5) centre (-235, -30) ccw
  arc A176 (-55, -332.5) -> (-55, -327.5) centre (-55, -330) ccw
  line L180 (-55, -332.5) -> (-65, -332.5)
  arc A177 (-65, -327.5) -> (-65, -332.5) centre (-65, -330) ccw
  line L181 (-65, -327.5) -> (-55, -327.5)
  arc A178 (-15, -12.5) -> (-15, -7.5) centre (-15, -10) ccw
  line L182 (-15, -12.5) -> (-25, -12.5)
  arc A179 (-25, -7.5) -> (-25, -12.5) centre (-25, -10) ccw
  line L183 (-25, -7.5) -> (-15, -7.5)
  arc A180 (-55, -212.5) -> (-55, -207.5) centre (-55, -210) ccw
  line L184 (-55, -212.5) -> (-65, -212.5)
  arc A181 (-65, -207.5) -> (-65, -212.5) centre (-65, -210) ccw
  line L185 (-65, -207.5) -> (-55, -207.5)
  arc A182 (-135, -212.5) -> (-135, -207.5) centre (-135, -210) ccw
  line L186 (-135, -212.5) -> (-145, -212.5)
  arc A183 (-145, -207.5) -> (-145, -212.5) centre (-145, -210) ccw
  line L187 (-145, -207.5) -> (-135, -207.5)
  line L188 (-75, -152.5) -> (-85, -152.5)
  arc A184 (-85, -147.5) -> (-85, -152.5) centre (-85, -150) ccw
  line L189 (-85, -147.5) -> (-75, -147.5)
  arc A185 (-75, -152.5) -> (-75, -147.5) centre (-75, -150) ccw
  arc A186 (-215, -292.5) -> (-215, -287.5) centre (-215, -290) ccw
  line L190 (-215, -292.5) -> (-225, -292.5)
  arc A187 (-225, -287.5) -> (-225, -292.5) centre (-225, -290) ccw
  line L191 (-225, -287.5) -> (-215, -287.5)
  arc A188 (-255, -292.5) -> (-255, -287.5) centre (-255, -290) ccw
  line L192 (-255, -292.5) -> (-265, -292.5)
  arc A189 (-265, -287.5) -> (-265, -292.5) centre (-265, -290) ccw
  line L193 (-265, -287.5) -> (-255, -287.5)
  line L194 (-195, -272.5) -> (-205, -272.5)